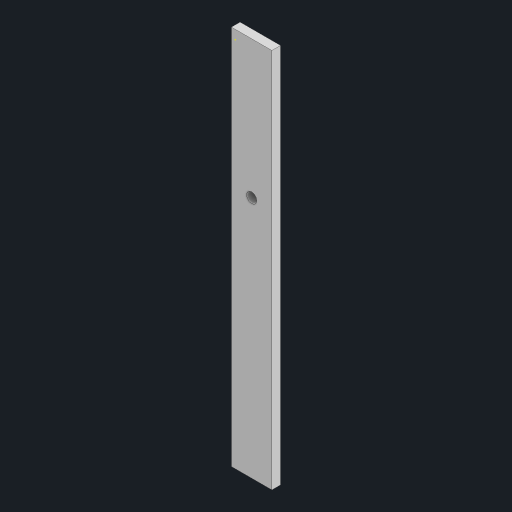
# Autodesk Inventor part: pillar
Saved by Autodesk Inventor 2024 (Build 280153000, 153)
## iProperties
Created: 2023-11-07
Part Number: pillar
Material: Generic
Document SubType Name: Modeling
Designer: 91840
Density: 1 g/cm^3
Appearance: Default
Author: 91840
Autodesk Inventor part; units mm, degrees
ref_plane "YZ Plane" through (0, 0, 0) normal (1, 0, 0) x (0, 1, 0)
ref_plane "XZ Plane" through (0, 0, 0) normal (0, 1, 0) x (-1, 0, 0)
ref_plane "XY Plane" through (0, 0, 0) normal (0, 0, 1) x (1, 0, 0)
sketch "Sketch1" plane through (0, 0, 0) normal (0, 0, 1) x (1, 0, 0)
  line L0 (-5, 11) -> (45, 11)
  line L1 (45, 11) -> (45, -459)
  line L2 (45, -459) -> (-5, -459)
  line L3 (-5, -459) -> (-5, 11)
  point P0 (0, 0)
  dimension "d0" = 50
  dimension "d1" = 470
  constraints: 8 end point, 2 parallel, 1 horizontal, 1 perpendicular
  measures "d0" distance of L1.end L2.end
  measures "d1" distance of L0.end L1.end
extrude "Extrusion1" add sketch "Sketch1" along normal blind 10.7
sketch "Sketch2" plane through (0, 0, 10.7) normal (0, 0, 1) x (1, 0, 0)
  point P0 (0, 0)
sketch "Sketch3" plane through (0, 0, 10.7) normal (0, 0, 1) x (1, 0, 0)
  circle A0 centre (20, -159) radius 6.35
  point P0 (0, 0)
  dimension "d4" = 12.7
  constraints: 1 centre point
  measures "d4" diameter of A0
extrude "Extrusion2" cut sketch "Sketch3" against normal through all
body "Solid1"
